Autodesk Inventor part; units mm, degrees
(part 2 of 2)
  spline S140 degree 2 poles (21.6159, 52.912) (21.6159, 52.7897) (21.701, 52.6195) (21.8632, 52.5397) (21.9616, 52.5397) knots 0 0 0 1 2 3 3 3
  spline S141 degree 2 poles (21.9616, 52.5397) (22.0308, 52.5397) (22.1611, 52.5849) (22.2675, 52.67) (22.3366, 52.7817) (22.3685, 52.8854) (22.3845, 52.9785) knots 0 0 0 1 2 3 4 5 5 5
  spline S142 degree 2 poles (52.1298, 59.6223) (52.0793, 59.0931) (52.0607, 58.7739) knots 0 0 0 1 1 1
  spline S143 degree 2 poles (52.0607, 58.7739) (52.0314, 58.3006) (52.0048, 57.548) knots 0 0 0 1 1 1
  spline S144 degree 2 poles (52.0048, 57.548) (51.9835, 56.9735) (51.9835, 56.7235) knots 0 0 0 1 1 1
  line L31 (51.9835, 56.7235) -> (51.9835, 56.4523)
  spline S145 degree 2 poles (51.9835, 56.4523) (51.7123, 56.4603) (51.5155, 56.4603) knots 0 0 0 1 1 1
  spline S146 degree 2 poles (51.5155, 56.4603) (51.324, 56.4603) (50.707, 56.439) (50.4358, 56.439) knots 0 0 0 1 2 2 2
  spline S147 degree 2 poles (50.4358, 56.439) (50.1246, 56.439) (49.6539, 56.5135) (49.247, 56.7448) (48.9731, 57.1198) (48.8295, 57.6251) (48.8295, 57.891) knots 0 0 0 1 2 3 4 5 5 5
  spline S148 degree 2 poles (48.8295, 57.891) (48.8295, 58.1543) (48.9412, 58.641) (49.1406, 59.0292) (49.4066, 59.3111) (49.5794, 59.4122) knots 0 0 0 1 2 3 4 4 4
  spline S149 degree 2 poles (49.5794, 59.4122) (49.7071, 59.484) (49.9677, 59.5691) (50.1938, 59.5957) knots 0 0 0 1 2 2 2
  spline S150 degree 2 poles (50.1938, 59.5957) (50.4438, 59.6223) (50.7629, 59.6223) knots 0 0 0 1 1 1
  line L32 (50.7629, 59.6223) -> (51.699, 59.6143)
  spline S151 degree 2 poles (51.699, 59.6143) (51.832, 59.6143) (52.1298, 59.6223) knots 0 0 0 1 1 1
  spline S152 degree 2 poles (51.1246, 58.9229) (50.9969, 58.9335) (50.8586, 58.9335) knots 0 0 0 1 1 1
  spline S153 degree 2 poles (50.8586, 58.9335) (50.6219, 58.9335) (50.2496, 58.8511) (49.9704, 58.5771) (49.8347, 58.1463) (49.8347, 57.9229) knots 0 0 0 1 2 3 4 4 4
  spline S154 degree 2 poles (49.8347, 57.9229) (49.8347, 57.6464) (50.0342, 57.2687) (50.3666, 57.1198) (50.6512, 57.1198) knots 0 0 0 1 2 3 3 3
  spline S155 degree 2 poles (50.6512, 57.1198) (50.8187, 57.1198) (51.0474, 57.1331) knots 0 0 0 1 1 1
  line L33 (51.0474, 57.1331) -> (51.1246, 58.9229)
  spline S156 degree 2 poles (46.1861, 58.9229) (46.2153, 59.0612) (46.3031, 59.5957) knots 0 0 0 1 1 1
  spline S157 degree 2 poles (46.3031, 59.5957) (46.5717, 59.6489) (46.9387, 59.6835) (47.1275, 59.6835) knots 0 0 0 1 2 2 2
  spline S158 degree 2 poles (47.1275, 59.6835) (47.4041, 59.6835) (47.8668, 59.6063) (48.2045, 59.4122) (48.4306, 59.1223) (48.5503, 58.7234) (48.5503, 58.5107) knots 0 0 0 1 2 3 4 5 5 5
  spline S159 degree 2 poles (48.5503, 58.5107) (48.5503, 58.2155) (48.3136, 57.6464) (47.9386, 57.3272) (47.4519, 57.1916) (47.1966, 57.1916) knots 0 0 0 1 2 3 4 4 4
  spline S160 degree 2 poles (47.1966, 57.1916) (46.9333, 57.1916) (46.452, 57.3139) (46.1169, 57.6198) (45.976, 58.0054) (45.976, 58.2288) knots 0 0 0 1 2 3 4 4 4
  spline S161 degree 2 poles (45.976, 58.2288) (45.976, 58.3617) (46.0052, 58.524) knots 0 0 0 1 1 1
  line L34 (46.0052, 58.524) -> (47.6328, 58.5266)
  spline S162 degree 2 poles (47.6328, 58.5266) (47.6354, 58.5639) (47.6354, 58.5931) knots 0 0 0 1 1 1
  spline S163 degree 2 poles (47.6354, 58.5931) (47.6354, 58.8431) (47.2764, 59.0798) (47.0211, 59.0798) knots 0 0 0 1 2 2 2
  spline S164 degree 2 poles (47.0211, 59.0798) (46.8669, 59.0798) (46.4733, 59.008) (46.1861, 58.9229) knots 0 0 0 1 2 2 2
  line L35 (47.6142, 58.1703) -> (46.8482, 58.1703)
  spline S165 degree 2 poles (46.8482, 58.1703) (46.8456, 58.1304) (46.8456, 58.1038) knots 0 0 0 1 1 1
  spline S166 degree 2 poles (46.8456, 58.1038) (46.8456, 57.9814) (46.9307, 57.8112) (47.0929, 57.7315) (47.1913, 57.7315) knots 0 0 0 1 2 3 3 3
  spline S167 degree 2 poles (47.1913, 57.7315) (47.2605, 57.7315) (47.3908, 57.7767) (47.4971, 57.8618) (47.5663, 57.9735) (47.5982, 58.0772) (47.6142, 58.1703) knots 0 0 0 1 2 3 4 5 5 5
  line L36 (45.0319, 59.6223) -> (45.2765, 58.8617)
  line L37 (45.2765, 58.8617) -> (45.8324, 57.2528)
  spline S168 degree 2 poles (45.8324, 57.2528) (45.5664, 57.2581) (45.3404, 57.2581) knots 0 0 0 1 1 1
  spline S169 degree 2 poles (45.3404, 57.2581) (45.1037, 57.2581) (44.8936, 57.2528) knots 0 0 0 1 1 1
  spline S170 degree 2 poles (44.8936, 57.2528) (44.8537, 57.4123) (44.6223, 58.2128) (44.4814, 58.766) knots 0 0 0 1 2 2 2
  line L38 (44.4814, 58.766) -> (44.4229, 58.5745)
  spline S171 degree 2 poles (44.4229, 58.5745) (44.4096, 58.5373) (44.3138, 58.2766) knots 0 0 0 1 1 1
  line L39 (44.3138, 58.2766) -> (43.9442, 57.2528)
  spline S172 degree 2 poles (43.9442, 57.2528) (43.6942, 57.2581) (43.4708, 57.2581) knots 0 0 0 1 1 1
  spline S173 degree 2 poles (43.4708, 57.2581) (43.2394, 57.2581) (42.9921, 57.2528) knots 0 0 0 1 1 1
  line L40 (42.9921, 57.2528) -> (43.3113, 57.9416)
  line L41 (43.3113, 57.9416) -> (43.9096, 59.3111)
  line L42 (43.9096, 59.3111) -> (44.0373, 59.6223)
  spline S174 degree 2 poles (44.0373, 59.6223) (44.3112, 59.617) (44.5213, 59.617) knots 0 0 0 1 1 1
  spline S175 degree 2 poles (44.5213, 59.617) (44.7473, 59.617) (45.0319, 59.6223) knots 0 0 0 1 1 1
  spline S176 degree 2 poles (40.5694, 58.9229) (40.5987, 59.0612) (40.6864, 59.5957) knots 0 0 0 1 1 1
  spline S177 degree 2 poles (40.6864, 59.5957) (40.955, 59.6489) (41.322, 59.6835) (41.5108, 59.6835) knots 0 0 0 1 2 2 2
  spline S178 degree 2 poles (41.5108, 59.6835) (41.7874, 59.6835) (42.2502, 59.6063) (42.5879, 59.4122) (42.8139, 59.1223) (42.9336, 58.7234) (42.9336, 58.5107) knots 0 0 0 1 2 3 4 5 5 5
  spline S179 degree 2 poles (42.9336, 58.5107) (42.9336, 58.2155) (42.6969, 57.6464) (42.322, 57.3272) (41.8353, 57.1916) (41.58, 57.1916) knots 0 0 0 1 2 3 4 4 4
  spline S180 degree 2 poles (41.58, 57.1916) (41.3167, 57.1916) (40.8354, 57.3139) (40.5003, 57.6198) (40.3593, 58.0054) (40.3593, 58.2288) knots 0 0 0 1 2 3 4 4 4
  spline S181 degree 2 poles (40.3593, 58.2288) (40.3593, 58.3617) (40.3886, 58.524) knots 0 0 0 1 1 1
  line L43 (40.3886, 58.524) -> (42.0161, 58.5266)
  spline S182 degree 2 poles (42.0161, 58.5266) (42.0188, 58.5639) (42.0188, 58.5931) knots 0 0 0 1 1 1
  spline S183 degree 2 poles (42.0188, 58.5931) (42.0188, 58.8431) (41.6598, 59.0798) (41.4045, 59.0798) knots 0 0 0 1 2 2 2
  spline S184 degree 2 poles (41.4045, 59.0798) (41.2502, 59.0798) (40.8566, 59.008) (40.5694, 58.9229) knots 0 0 0 1 2 2 2
  line L44 (41.9975, 58.1703) -> (41.2316, 58.1703)
  spline S185 degree 2 poles (41.2316, 58.1703) (41.2289, 58.1304) (41.2289, 58.1038) knots 0 0 0 1 1 1
  spline S186 degree 2 poles (41.2289, 58.1038) (41.2289, 57.9814) (41.314, 57.8112) (41.4763, 57.7315) (41.5747, 57.7315) knots 0 0 0 1 2 3 3 3
  spline S187 degree 2 poles (41.5747, 57.7315) (41.6438, 57.7315) (41.7741, 57.7767) (41.8805, 57.8618) (41.9496, 57.9735) (41.9816, 58.0772) (41.9975, 58.1703) knots 0 0 0 1 2 3 4 5 5 5
  line L45 (40.0588, 59.6223) -> (40.0163, 59.1223)
  line L46 (40.0163, 59.1223) -> (39.9285, 57.3857)
  line L47 (39.9285, 57.3857) -> (39.9019, 56.4523)
  spline S188 degree 2 poles (39.9019, 56.4523) (39.5801, 56.4576) (39.4179, 56.4576) knots 0 0 0 1 1 1
  spline S189 degree 2 poles (39.4179, 56.4576) (39.2051, 56.4576) (38.9498, 56.4523) knots 0 0 0 1 1 1
  line L48 (38.9498, 56.4523) -> (39.003, 57.165)
  line L49 (39.003, 57.165) -> (39.0881, 58.9202)
  line L50 (39.0881, 58.9202) -> (39.1067, 59.6223)
  spline S190 degree 2 poles (39.1067, 59.6223) (39.3541, 59.6196) (39.5535, 59.6196) knots 0 0 0 1 1 1
  line L51 (39.5535, 59.6196) -> (40.0588, 59.6223)
  spline S191 degree 2 poles (37.2, 57.1916) (36.9127, 57.1916) (36.3809, 57.3671) (36.0139, 57.6995) (35.8383, 58.1437) (35.8383, 58.399) knots 0 0 0 1 2 3 4 4 4
  spline S192 degree 2 poles (35.8383, 58.399) (35.8383, 58.649) (35.9953, 59.0957) (36.3649, 59.4893) (36.9393, 59.6835) (37.2611, 59.6835) knots 0 0 0 1 2 3 4 4 4
  spline S193 degree 2 poles (37.2611, 59.6835) (37.5537, 59.6835) (38.0988, 59.5106) (38.4632, 59.1808) (38.6467, 58.7208) (38.6467, 58.4681) knots 0 0 0 1 2 3 4 4 4
  spline S194 degree 2 poles (38.6467, 58.4681) (38.6467, 58.2155) (38.4685, 57.7554) (38.0802, 57.3884) (37.5084, 57.1916) (37.2, 57.1916) knots 0 0 0 1 2 3 4 4 4
  spline S195 degree 2 poles (37.2159, 57.8751) (37.3648, 57.8751) (37.5962, 58.0293) (37.7159, 58.3218) (37.7159, 58.4974) knots 0 0 0 1 2 3 3 3
  spline S196 degree 2 poles (37.7159, 58.4974) (37.7159, 58.7527) (37.4606, 59.0239) (37.2664, 59.0239) knots 0 0 0 1 2 2 2
  spline S197 degree 2 poles (37.2664, 59.0239) (37.1202, 59.0239) (36.8888, 58.8697) (36.7691, 58.5639) (36.7691, 58.391) knots 0 0 0 1 2 3 3 3
  spline S198 degree 2 poles (36.7691, 58.391) (36.7691, 58.2474) (36.8622, 58.0134) (37.075, 57.8751) (37.2159, 57.8751) knots 0 0 0 1 2 3 3 3
  spline S199 degree 2 poles (35.5644, 60.71) (35.5219, 60.234) (35.4926, 59.7606) knots 0 0 0 1 1 1
  spline S200 degree 2 poles (35.4926, 59.7606) (35.4394, 58.9495) (35.3995, 57.8511) (35.3995, 57.3113) knots 0 0 0 1 2 2 2
  spline S201 degree 2 poles (35.3995, 57.3113) (34.9288, 57.2395) (34.3943, 57.1916) (34.1284, 57.1916) knots 0 0 0 1 2 2 2
  spline S202 degree 2 poles (34.1284, 57.1916) (33.7933, 57.1916) (33.2295, 57.3299) (32.8891, 57.6836) (32.7162, 58.1729) (32.7162, 58.4389) knots 0 0 0 1 2 3 4 4 4
  spline S203 degree 2 poles (32.7162, 58.4389) (32.7162, 58.6835) (32.8545, 59.1409) (33.1444, 59.5079) (33.5167, 59.6835) (33.7454, 59.6835) knots 0 0 0 1 2 3 4 4 4
  spline S204 degree 2 poles (33.7454, 59.6835) (33.8598, 59.6835) (34.1044, 59.6382) (34.3225, 59.5558) (34.4688, 59.4707) (34.5778, 59.3883) knots 0 0 0 1 2 3 4 4 4
  line L52 (34.5778, 59.3883) -> (34.6017, 60.0372)
  spline S205 degree 2 poles (34.6017, 60.0372) (34.6203, 60.4813) (34.6203, 60.71) knots 0 0 0 1 1 1
  spline S206 degree 2 poles (34.6203, 60.71) (34.8889, 60.7047) (35.0804, 60.7047) knots 0 0 0 1 1 1
  spline S207 degree 2 poles (35.0804, 60.7047) (35.248, 60.7047) (35.5644, 60.71) knots 0 0 0 1 1 1
  spline S208 degree 2 poles (34.4954, 57.9043) (34.514, 58.008) (34.5273, 58.141) (34.5432, 58.3671) (34.5432, 58.4335) knots 0 0 0 1 2 3 3 3
  spline S209 degree 2 poles (34.5432, 58.4335) (34.5432, 58.625) (34.4235, 58.883) (34.2108, 59.0239) (34.0911, 59.0239) knots 0 0 0 1 2 3 3 3
  spline S210 degree 2 poles (34.0911, 59.0239) (33.9635, 59.0239) (33.7481, 58.8777) (33.6231, 58.5851) (33.6231, 58.4016) knots 0 0 0 1 2 3 3 3
  spline S211 degree 2 poles (33.6231, 58.4016) (33.6231, 58.1543) (33.8864, 57.8511) (34.1363, 57.8511) knots 0 0 0 1 2 2 2
  spline S212 degree 2 poles (34.1363, 57.8511) (34.2959, 57.8511) (34.4954, 57.9043) knots 0 0 0 1 1 1
  spline S213 degree 2 poles (30.0754, 58.9229) (30.1047, 59.0612) (30.1925, 59.5957) knots 0 0 0 1 1 1
  spline S214 degree 2 poles (30.1925, 59.5957) (30.461, 59.6489) (30.828, 59.6835) (31.0169, 59.6835) knots 0 0 0 1 2 2 2
  spline S215 degree 2 poles (31.0169, 59.6835) (31.2934, 59.6835) (31.7562, 59.6063) (32.0939, 59.4122) (32.32, 59.1223) (32.4396, 58.7234) (32.4396, 58.5107) knots 0 0 0 1 2 3 4 5 5 5
  spline S216 degree 2 poles (32.4396, 58.5107) (32.4396, 58.2155) (32.203, 57.6464) (31.828, 57.3272) (31.3413, 57.1916) (31.086, 57.1916) knots 0 0 0 1 2 3 4 4 4
  spline S217 degree 2 poles (31.086, 57.1916) (30.8227, 57.1916) (30.3414, 57.3139) (30.0063, 57.6198) (29.8653, 58.0054) (29.8653, 58.2288) knots 0 0 0 1 2 3 4 4 4
  spline S218 degree 2 poles (29.8653, 58.2288) (29.8653, 58.3617) (29.8946, 58.524) knots 0 0 0 1 1 1
  line L53 (29.8946, 58.524) -> (31.5221, 58.5266)
  spline S219 degree 2 poles (31.5221, 58.5266) (31.5248, 58.5639) (31.5248, 58.5931) knots 0 0 0 1 1 1
  spline S220 degree 2 poles (31.5248, 58.5931) (31.5248, 58.8431) (31.1658, 59.0798) (30.9105, 59.0798) knots 0 0 0 1 2 2 2
  spline S221 degree 2 poles (30.9105, 59.0798) (30.7562, 59.0798) (30.3627, 59.008) (30.0754, 58.9229) knots 0 0 0 1 2 2 2
  line L54 (31.5035, 58.1703) -> (30.7376, 58.1703)
  spline S222 degree 2 poles (30.7376, 58.1703) (30.735, 58.1304) (30.735, 58.1038) knots 0 0 0 1 1 1
  spline S223 degree 2 poles (30.735, 58.1038) (30.735, 57.9814) (30.8201, 57.8112) (30.9823, 57.7315) (31.0807, 57.7315) knots 0 0 0 1 2 3 3 3
  spline S224 degree 2 poles (31.0807, 57.7315) (31.1498, 57.7315) (31.2801, 57.7767) (31.3865, 57.8618) (31.4557, 57.9735) (31.4876, 58.0772) (31.5035, 58.1703) knots 0 0 0 1 2 3 4 5 5 5
  spline S225 degree 2 poles (26.9453, 59.6223) (27.1927, 59.617) (27.3575, 59.617) knots 0 0 0 1 1 1
  spline S226 degree 2 poles (27.3575, 59.617) (27.5437, 59.617) (27.8096, 59.6223) knots 0 0 0 1 1 1
  line L55 (27.8096, 59.6223) -> (27.7963, 59.3271)
  spline S227 degree 2 poles (27.7963, 59.3271) (27.8868, 59.4175) (28.0197, 59.5266) (28.2325, 59.6276) (28.4771, 59.6835) (28.6075, 59.6835) knots 0 0 0 1 2 3 4 4 4
  spline S228 degree 2 poles (28.6075, 59.6835) (28.8282, 59.6835) (29.2165, 59.5212) (29.4904, 59.2207) (29.626, 58.8112) (29.626, 58.5904) knots 0 0 0 1 2 3 4 4 4
  spline S229 degree 2 poles (29.626, 58.5904) (29.626, 58.2766) (29.3787, 57.6783) (28.9824, 57.3325) (28.4825, 57.1916) (28.1926, 57.1916) knots 0 0 0 1 2 3 4 4 4
  spline S230 degree 2 poles (28.1926, 57.1916) (27.9984, 57.1916) (27.7405, 57.2262) knots 0 0 0 1 1 1
  spline S231 degree 2 poles (27.7405, 57.2262) (27.7219, 56.9496) (27.7139, 56.4523) knots 0 0 0 1 1 1
  spline S232 degree 2 poles (27.7139, 56.4523) (27.4293, 56.4576) (27.2485, 56.4576) knots 0 0 0 1 1 1
  spline S233 degree 2 poles (27.2485, 56.4576) (27.0145, 56.4576) (26.7751, 56.4523) knots 0 0 0 1 1 1
  spline S234 degree 2 poles (26.7751, 56.4523) (26.8416, 57.1411) (26.9453, 59.1303) (26.9453, 59.6223) knots 0 0 0 1 2 2 2
  spline S235 degree 2 poles (27.7724, 57.8299) (27.8947, 57.8033) (28.0064, 57.8033) knots 0 0 0 1 1 1
  spline S236 degree 2 poles (28.0064, 57.8033) (28.2325, 57.8033) (28.5489, 57.9761) (28.7191, 58.3458) (28.7191, 58.524) knots 0 0 0 1 2 3 3 3
  spline S237 degree 2 poles (28.7191, 58.524) (28.7191, 58.6596) (28.6234, 58.875) (28.424, 59) (28.3043, 59) knots 0 0 0 1 2 3 3 3
  spline S238 degree 2 poles (28.3043, 59) (28.1766, 59) (27.9639, 58.8564) (27.8309, 58.5771) (27.7804, 58.1942) (27.7724, 57.8299) knots 0 0 0 1 2 3 4 4 4
  spline S239 degree 2 poles (25.246, 59.6223) (25.1821, 58.891) (25.0838, 56.9443) (25.0838, 56.4523) knots 0 0 0 1 2 2 2
  spline S240 degree 2 poles (25.0838, 56.4523) (24.8152, 56.4576) (24.5785, 56.4576) knots 0 0 0 1 1 1
  spline S241 degree 2 poles (24.5785, 56.4576) (24.3498, 56.4576) (24.129, 56.4523) knots 0 0 0 1 1 1
  spline S242 degree 2 poles (24.129, 56.4523) (24.1796, 56.814) (24.2035, 57.2501) knots 0 0 0 1 1 1
  spline S243 degree 2 poles (24.2035, 57.2501) (23.9907, 57.2155) (23.762, 57.1916) (23.653, 57.1916) knots 0 0 0 1 2 2 2
  spline S244 degree 2 poles (23.653, 57.1916) (23.294, 57.1916) (22.786, 57.4177) (22.4669, 57.9522) (22.4669, 58.3378) knots 0 0 0 1 2 3 3 3
  spline S245 degree 2 poles (22.4669, 58.3378) (22.4669, 58.7208) (22.7701, 59.3696) (23.2754, 59.6835) (23.6131, 59.6835) knots 0 0 0 1 2 3 3 3
  spline S246 degree 2 poles (23.6131, 59.6835) (23.7381, 59.6835) (23.9668, 59.6329) (24.1503, 59.5319) (24.278, 59.4202) (24.3577, 59.3271) knots 0 0 0 1 2 3 4 4 4
  line L56 (24.3577, 59.3271) -> (24.3684, 59.6223)
  spline S247 degree 2 poles (24.3684, 59.6223) (24.6157, 59.617) (24.7832, 59.617) knots 0 0 0 1 1 1
  spline S248 degree 2 poles (24.7832, 59.617) (24.9215, 59.617) (25.246, 59.6223) knots 0 0 0 1 1 1
  spline S249 degree 2 poles (24.2673, 57.9017) (24.2833, 58.2873) (24.2833, 58.3724) knots 0 0 0 1 1 1
  spline S250 degree 2 poles (24.2833, 58.3724) (24.2833, 58.5904) (24.2061, 58.8457) (23.9907, 59) (23.8551, 59) knots 0 0 0 1 2 3 3 3
  spline S251 degree 2 poles (23.8551, 59) (23.7168, 59) (23.5067, 58.8457) (23.3977, 58.5532) (23.3977, 58.3883) knots 0 0 0 1 2 3 3 3
  spline S252 degree 2 poles (23.3977, 58.3883) (23.3977, 58.1463) (23.661, 57.8511) (23.9083, 57.8511) knots 0 0 0 1 2 2 2
  spline S253 degree 2 poles (23.9083, 57.8511) (24.0625, 57.8511) (24.2673, 57.9017) knots 0 0 0 1 1 1
  spline S254 degree 2 poles (22.3153, 60.6834) (22.3871, 60.1302) (22.4137, 59.9946) knots 0 0 0 1 1 1
  spline S255 degree 2 poles (22.4137, 59.9946) (22.2675, 60.0637) (22.0414, 60.1143) (21.9616, 60.1143) knots 0 0 0 1 2 2 2
  spline S256 degree 2 poles (21.9616, 60.1143) (21.8739, 60.1143) (21.7249, 60.0691) (21.6345, 59.9999) (21.5308, 59.8616) (21.4803, 59.7606) (21.4537, 59.6675) knots 0 0 0 1 2 3 4 5 5 5
  line L57 (21.4537, 59.6675) -> (21.8898, 58.3484)
  line L58 (21.8898, 58.3484) -> (22.2648, 57.2528)
  spline S257 degree 2 poles (22.2648, 57.2528) (21.9191, 57.2581) (21.7808, 57.2581) knots 0 0 0 1 1 1
  spline S258 degree 2 poles (21.7808, 57.2581) (21.6159, 57.2581) (21.3367, 57.2528) knots 0 0 0 1 1 1
  spline S259 degree 2 poles (21.3367, 57.2528) (21.2915, 57.4309) (21.0521, 58.3085) (20.9989, 58.5559) knots 0 0 0 1 2 2 2
  spline S260 degree 2 poles (20.9989, 58.5559) (20.9697, 58.6942) (20.9404, 58.9043) knots 0 0 0 1 1 1
  line L59 (20.9404, 58.9043) -> (20.8925, 58.7208)
  spline S261 degree 2 poles (20.8925, 58.7208) (20.8686, 58.6463) (20.8101, 58.4548) (20.7622, 58.3218) knots 0 0 0 1 2 2 2
  line L60 (20.7622, 58.3218) -> (20.6106, 57.899)
  line L61 (20.6106, 57.899) -> (20.3607, 57.2528)
  spline S262 degree 2 poles (20.3607, 57.2528) (20.0708, 57.2581) (19.9219, 57.2581) knots 0 0 0 1 1 1
  spline S263 degree 2 poles (19.9219, 57.2581) (19.7916, 57.2581) (19.4565, 57.2528) knots 0 0 0 1 1 1
  line L62 (19.4565, 57.2528) -> (19.9059, 58.2633)
  line L63 (19.9059, 58.2633) -> (20.717, 60.1409)
  spline S264 degree 2 poles (20.717, 60.1409) (20.7941, 60.3004) (20.8659, 60.3935) knots 0 0 0 1 1 1
  spline S265 degree 2 poles (20.8659, 60.3935) (20.9351, 60.476) (21.0122, 60.5398) knots 0 0 0 1 1 1
  spline S266 degree 2 poles (21.0122, 60.5398) (21.0867, 60.5983) (21.1744, 60.6355) knots 0 0 0 1 1 1
  spline S267 degree 2 poles (21.1744, 60.6355) (21.2888, 60.6887) (21.4297, 60.7206) knots 0 0 0 1 1 1
  spline S268 degree 2 poles (21.4297, 60.7206) (21.5813, 60.7525) (21.7409, 60.7525) knots 0 0 0 1 1 1
  spline S269 degree 2 poles (21.7409, 60.7525) (21.8127, 60.7525) (22.0494, 60.7313) (22.1956, 60.71) (22.3153, 60.6834) knots 0 0 0 1 2 3 3 3
  spline S270 degree 2 poles (19.2889, 59.6223) (19.2703, 59.3111) (19.257, 58.7819) knots 0 0 0 1 1 1
  line L64 (19.257, 58.7819) -> (18.7783, 58.7899)
  spline S271 degree 2 poles (18.7783, 58.7899) (18.7012, 58.7899) (18.3741, 58.7819) knots 0 0 0 1 1 1
  spline S272 degree 2 poles (18.3741, 58.7819) (18.3927, 59.0346) (18.4166, 59.6223) knots 0 0 0 1 1 1
  line L65 (18.4166, 59.6223) -> (18.8209, 59.617)
  spline S273 degree 2 poles (18.8209, 59.617) (18.8634, 59.617) (19.2889, 59.6223) knots 0 0 0 1 1 1
  spline S274 degree 2 poles (19.2331, 58.0931) (19.2118, 57.7208) (19.1985, 57.2528) knots 0 0 0 1 1 1
  line L66 (19.1985, 57.2528) -> (18.7225, 57.2581)
  spline S275 degree 2 poles (18.7225, 57.2581) (18.6454, 57.2581) (18.3182, 57.2528) knots 0 0 0 1 1 1
  spline S276 degree 2 poles (18.3182, 57.2528) (18.3342, 57.4788) (18.3608, 58.0931) knots 0 0 0 1 1 1
  line L67 (18.3608, 58.0931) -> (18.765, 58.0852)
  spline S277 degree 2 poles (18.765, 58.0852) (18.8076, 58.0852) (19.2331, 58.0931) knots 0 0 0 1 1 1
  spline S278 degree 2 poles (50.1326, 63.1972) (50.1326, 63.3753) (50.3081, 63.6865) (50.614, 63.862) (50.7868, 63.862) knots 0 0 0 1 2 3 3 3
  spline S279 degree 2 poles (50.7868, 63.862) (50.9597, 63.862) (51.2655, 63.6838) (51.441, 63.3727) (51.441, 63.1972) knots 0 0 0 1 2 3 3 3
  spline S280 degree 2 poles (51.441, 63.1972) (51.441, 63.0216) (51.2655, 62.7131) (50.9597, 62.535) (50.7815, 62.535) knots 0 0 0 1 2 3 3 3
  spline S281 degree 2 poles (50.7815, 62.535) (50.6113, 62.535) (50.3081, 62.7105) (50.1326, 63.019) (50.1326, 63.1972) knots 0 0 0 1 2 3 3 3
  line L68 (43.04, 64.8141) -> (42.8485, 64.479)
  line L69 (42.8485, 64.479) -> (41.6465, 62.2185)
  line L70 (41.6465, 62.2185) -> (41.5188, 61.9659)
  spline S282 degree 2 poles (41.5188, 61.9659) (41.463, 61.8542) (41.3646, 61.6441) knots 0 0 0 1 1 1
  spline S283 degree 2 poles (41.3646, 61.6441) (40.955, 61.6494) (40.7662, 61.6494) knots 0 0 0 1 1 1
  spline S284 degree 2 poles (40.7662, 61.6494) (40.4391, 61.6494) (40.1599, 61.6441) knots 0 0 0 1 1 1
  line L71 (40.1599, 61.6441) -> (39.8221, 62.6121)
  line L72 (39.8221, 62.6121) -> (39.1333, 64.4737)
  line L73 (39.1333, 64.4737) -> (38.9977, 64.8141)
  spline S285 degree 2 poles (38.9977, 64.8141) (39.3993, 64.8087) (39.4844, 64.8087) knots 0 0 0 1 1 1
  spline S286 degree 2 poles (39.4844, 64.8087) (39.6812, 64.8087) (40.0588, 64.8141) knots 0 0 0 1 1 1
  spline S287 degree 2 poles (40.0588, 64.8141) (40.1599, 64.4311) (40.354, 63.9125) knots 0 0 0 1 1 1
  line L74 (40.354, 63.9125) -> (41.5241, 63.9125)
  spline S288 degree 2 poles (41.5241, 63.9125) (41.7236, 64.3221) (41.9417, 64.8141) knots 0 0 0 1 1 1
  spline S289 degree 2 poles (41.9417, 64.8141) (42.3725, 64.8087) (42.4709, 64.8087) knots 0 0 0 1 1 1
  spline S290 degree 2 poles (42.4709, 64.8087) (42.6464, 64.8087) (43.04, 64.8141) knots 0 0 0 1 1 1
  line L75 (41.2422, 63.237) -> (40.5215, 63.237)
  spline S291 degree 2 poles (40.5215, 63.237) (40.7901, 62.418) (40.8141, 62.3355) knots 0 0 0 1 1 1
  spline S292 degree 2 poles (40.8141, 62.3355) (40.9683, 62.6759) (41.0747, 62.894) knots 0 0 0 1 1 1
  line L76 (41.0747, 62.894) -> (41.2422, 63.237)
  line L77 (38.7876, 64.8141) -> (38.7451, 64.3141)
  line L78 (38.7451, 64.3141) -> (38.6573, 62.5775)
  line L79 (38.6573, 62.5775) -> (38.6307, 61.6441)
  spline S293 degree 2 poles (38.6307, 61.6441) (38.3089, 61.6494) (38.1467, 61.6494) knots 0 0 0 1 1 1
  spline S294 degree 2 poles (38.1467, 61.6494) (37.934, 61.6494) (37.6786, 61.6441) knots 0 0 0 1 1 1
  line L80 (37.6786, 61.6441) -> (37.7318, 62.3568)
  line L81 (37.7318, 62.3568) -> (37.8169, 64.112)
  line L82 (37.8169, 64.112) -> (37.8356, 64.8141)
  spline S295 degree 2 poles (37.8356, 64.8141) (38.0829, 64.8114) (38.2823, 64.8114) knots 0 0 0 1 1 1
  line L83 (38.2823, 64.8114) -> (38.7876, 64.8141)
  spline S296 degree 2 poles (37.2053, 64.8141) (37.1601, 64.3673) (37.0989, 63.1094) knots 0 0 0 1 1 1
  line L84 (37.0989, 63.1094) -> (37.3808, 63.1094)
  spline S297 degree 2 poles (37.3808, 63.1094) (37.3728, 63.0376) (37.3489, 62.5669) (37.3462, 62.4632) knots 0 0 0 1 2 2 2
  line L85 (37.3462, 62.4632) -> (37.0191, 62.4632)
  spline S298 degree 2 poles (37.0191, 62.4632) (37.0218, 62.3701) (37.0218, 62.3036) knots 0 0 0 1 1 1
  spline S299 degree 2 poles (37.0218, 62.3036) (37.0218, 62.0908) (36.9766, 61.8488) (36.8596, 61.6786) (36.6441, 61.5457) (36.3702, 61.5005) (36.224, 61.5005) knots 0 0 0 1 2 3 4 5 5 5
  spline S300 degree 2 poles (36.224, 61.5005) (36.091, 61.5005) (35.7772, 61.535) (35.5565, 61.5935) knots 0 0 0 1 2 2 2
  spline S301 degree 2 poles (35.5565, 61.5935) (35.5511, 61.9632) (35.5272, 62.2052) knots 0 0 0 1 1 1
  spline S302 degree 2 poles (35.5272, 62.2052) (35.7586, 62.1228) (35.9421, 62.1228) knots 0 0 0 1 1 1
  spline S303 degree 2 poles (35.9421, 62.1228) (36.0671, 62.1228) (36.2107, 62.2398) (36.2107, 62.394) knots 0 0 0 1 2 2 2
  line L86 (36.2107, 62.394) -> (36.208, 62.4632)
  line L87 (36.208, 62.4632) -> (35.6708, 62.4632)
  spline S304 degree 2 poles (35.6708, 62.4632) (35.6894, 62.7318) (35.708, 63.1094) knots 0 0 0 1 1 1
  line L88 (35.708, 63.1094) -> (36.1894, 63.1094)
  line L89 (36.1894, 63.1094) -> (36.2665, 64.8141)
  spline S305 degree 2 poles (36.2665, 64.8141) (36.5431, 64.8087) (36.7399, 64.8087) knots 0 0 0 1 1 1
  spline S306 degree 2 poles (36.7399, 64.8087) (36.9393, 64.8087) (37.2053, 64.8141) knots 0 0 0 1 1 1
  spline S307 degree 2 poles (35.2081, 63.12) (35.1629, 62.8887) (35.1416, 62.7158) (35.115, 62.5296) knots 0 0 0 1 2 2 2
  spline S308 degree 2 poles (35.115, 62.5296) (34.4475, 62.3834) (33.9661, 62.3834) knots 0 0 0 1 1 1
  spline S309 degree 2 poles (33.9661, 62.3834) (33.6922, 62.3834) (33.2375, 62.5057) (32.9822, 62.7796) (32.9822, 63.0349) knots 0 0 0 1 2 3 3 3
  spline S310 degree 2 poles (32.9822, 63.0349) (32.9822, 63.1652) (33.0513, 64.0748) (33.0699, 64.8141) knots 0 0 0 1 2 2 2
  spline S311 degree 2 poles (33.0699, 64.8141) (33.296, 64.8087) (33.522, 64.8087) knots 0 0 0 1 1 1
  spline S312 degree 2 poles (33.522, 64.8087) (33.7401, 64.8087) (33.9874, 64.8141) knots 0 0 0 1 1 1
  spline S313 degree 2 poles (33.9874, 64.8141) (33.9555, 64.5588) (33.9156, 63.7609) knots 0 0 0 1 1 1
  spline S314 degree 2 poles (33.9156, 63.7609) (34.0034, 63.8035) (34.1044, 63.8407) (34.3544, 63.9152) (34.4954, 63.9657) (34.5991, 64.0455) (34.6443, 64.1279) (34.6443, 64.1785) knots 0 0 0 1 2 3 4 5 6 6 6
  spline S315 degree 2 poles (34.6443, 64.1785) (34.6443, 64.2583) (34.5193, 64.3699) (34.3837, 64.3699) knots 0 0 0 1 2 2 2
  spline S316 degree 2 poles (34.3837, 64.3699) (34.3331, 64.3699) (34.2241, 64.354) (34.1257, 64.3221) knots 0 0 0 1 2 2 2
  spline S317 degree 2 poles (34.1257, 64.3221) (34.1922, 64.5003) (34.2853, 64.8433) knots 0 0 0 1 1 1
  spline S318 degree 2 poles (34.2853, 64.8433) (34.4847, 64.8752) (34.6629, 64.8752) knots 0 0 0 1 1 1
  spline S319 degree 2 poles (34.6629, 64.8752) (34.9501, 64.8752) (35.3331, 64.7157) (35.5405, 64.3566) (35.5405, 64.1785) knots 0 0 0 1 2 3 3 3
  spline S320 degree 2 poles (35.5405, 64.1785) (35.5405, 64.0694) (35.4634, 63.8593) (35.3011, 63.6599) (35.0831, 63.5189) (34.7054, 63.3939) (34.4156, 63.3381) knots 0 0 0 1 2 3 4 5 5 5
  spline S321 degree 2 poles (34.4156, 63.3381) (34.2932, 63.3142) (34.0911, 63.261) (34.006, 63.2211) (33.9528, 63.1679) (33.9289, 63.1094) (33.9289, 63.0775) knots 0 0 0 1 2 3 4 5 5 5
  spline S322 degree 2 poles (33.9289, 63.0775) (33.9289, 62.9897) (34.0778, 62.894) (34.2214, 62.894) knots 0 0 0 1 2 2 2
  spline S323 degree 2 poles (34.2214, 62.894) (34.6203, 62.894) (35.2081, 63.12) knots 0 0 0 1 1 1
  spline S324 degree 2 poles (32.57, 64.8141) (32.5035, 64.2875) (32.4317, 63.0137) (32.4237, 62.4445) knots 0 0 0 1 2 2 2
  spline S325 degree 2 poles (32.4237, 62.4445) (32.1471, 62.4499) (31.945, 62.4499) knots 0 0 0 1 1 1
  spline S326 degree 2 poles (31.945, 62.4499) (31.7083, 62.4499) (31.4929, 62.4445) knots 0 0 0 1 1 1
  line L90 (31.4929, 62.4445) -> (31.5168, 62.761)
  spline S327 degree 2 poles (31.5168, 62.761) (31.4397, 62.6733) (31.328, 62.5749) (31.1631, 62.4791) (30.977, 62.418) (30.7562, 62.3834) (30.6366, 62.3834) knots 0 0 0 1 2 3 4 5 5 5
  spline S328 degree 2 poles (30.6366, 62.3834) (30.469, 62.3834) (30.1499, 62.4552) (29.9371, 62.5882) (29.7909, 62.7849) (29.7457, 63.0137) (29.7457, 63.1333) knots 0 0 0 1 2 3 4 5 5 5
  spline S329 degree 2 poles (29.7457, 63.1333) (29.7457, 63.2211) (29.7643, 63.5136) knots 0 0 0 1 1 1
  line L91 (29.7643, 63.5136) -> (29.8042, 64.354)
  spline S330 degree 2 poles (29.8042, 64.354) (29.8148, 64.604) (29.8148, 64.8141) knots 0 0 0 1 1 1
  spline S331 degree 2 poles (29.8148, 64.8141) (30.0515, 64.8087) (30.2536, 64.8087) knots 0 0 0 1 1 1
  spline S332 degree 2 poles (30.2536, 64.8087) (30.5302, 64.8087) (30.7589, 64.8141) knots 0 0 0 1 1 1
  spline S333 degree 2 poles (30.7589, 64.8141) (30.7376, 64.604) (30.6924, 63.7689) (30.6924, 63.6014) knots 0 0 0 1 2 2 2
  spline S334 degree 2 poles (30.6924, 63.6014) (30.6924, 63.3381) (30.8945, 63.1307) (31.0461, 63.1307) knots 0 0 0 1 2 2 2
  spline S335 degree 2 poles (31.0461, 63.1307) (31.1817, 63.1307) (31.4211, 63.3062) (31.5514, 63.6439) (31.6046, 64.4152) (31.6126, 64.8141) knots 0 0 0 1 2 3 4 4 4
  spline S336 degree 2 poles (31.6126, 64.8141) (31.8466, 64.8087) (32.0673, 64.8087) knots 0 0 0 1 1 1
  spline S337 degree 2 poles (32.0673, 64.8087) (32.2987, 64.8087) (32.57, 64.8141) knots 0 0 0 1 1 1
  spline S338 degree 2 poles (27.9346, 62.3834) (27.6474, 62.3834) (27.1155, 62.5589) (26.7485, 62.8913) (26.573, 63.3354) (26.573, 63.5907) knots 0 0 0 1 2 3 4 4 4
  spline S339 degree 2 poles (26.573, 63.5907) (26.573, 63.8407) (26.7299, 64.2875) (27.0996, 64.6811) (27.674, 64.8752) (27.9958, 64.8752) knots 0 0 0 1 2 3 4 4 4
  spline S340 degree 2 poles (27.9958, 64.8752) (28.2883, 64.8752) (28.8335, 64.7024) (29.1978, 64.3726) (29.3813, 63.9125) (29.3813, 63.6599) knots 0 0 0 1 2 3 4 4 4
  spline S341 degree 2 poles (29.3813, 63.6599) (29.3813, 63.4072) (29.2032, 62.9472) (28.8149, 62.5802) (28.2431, 62.3834) (27.9346, 62.3834) knots 0 0 0 1 2 3 4 4 4
  spline S342 degree 2 poles (27.9506, 63.0668) (28.0995, 63.0668) (28.3309, 63.2211) (28.4505, 63.5136) (28.4505, 63.6891) knots 0 0 0 1 2 3 3 3
  spline S343 degree 2 poles (28.4505, 63.6891) (28.4505, 63.9444) (28.1952, 64.2157) (28.0011, 64.2157) knots 0 0 0 1 2 2 2
  spline S344 degree 2 poles (28.0011, 64.2157) (27.8548, 64.2157) (27.6235, 64.0615) (27.5038, 63.7556) (27.5038, 63.5828) knots 0 0 0 1 2 3 3 3
  spline S345 degree 2 poles (27.5038, 63.5828) (27.5038, 63.4392) (27.5969, 63.2051) (27.8096, 63.0668) (27.9506, 63.0668) knots 0 0 0 1 2 3 3 3
  spline S346 degree 2 poles (25.0173, 64.8141) (24.9588, 64.2157) (24.9056, 63.4072) (24.8524, 62.0669) (24.8524, 61.8488) knots 0 0 0 1 2 3 3 3
  line L92 (24.8524, 61.8488) -> (24.855, 61.6441)
  spline S347 degree 2 poles (24.855, 61.6441) (24.3072, 61.6494) (23.528, 61.6494) knots 0 0 0 1 1 1
  spline S348 degree 2 poles (23.528, 61.6494) (22.81, 61.6494) (22.2621, 61.6441) knots 0 0 0 1 1 1
  line L93 (22.2621, 61.6441) -> (22.2675, 61.7212)
  spline S349 degree 2 poles (22.2675, 61.7212) (22.2701, 61.7478) (22.2781, 61.9206) knots 0 0 0 1 1 1
  line L94 (22.2781, 61.9206) -> (22.2914, 62.1733)
  spline S350 degree 2 poles (22.2914, 62.1733) (22.2967, 62.2531) (22.2967, 62.3382) knots 0 0 0 1 1 1
  spline S351 degree 2 poles (22.2967, 62.3382) (22.7461, 62.3196) (23.0493, 62.3196) knots 0 0 0 1 1 1
  spline S352 degree 2 poles (23.0493, 62.3196) (23.3844, 62.3196) (23.6184, 62.3222) (23.8684, 62.3302) knots 0 0 0 1 2 2 2
  line L95 (23.8684, 62.3302) -> (23.8977, 62.8647)
  spline S353 degree 2 poles (23.8977, 62.8647) (23.6237, 62.8727) (23.2567, 62.8727) knots 0 0 0 1 1 1
  spline S354 degree 2 poles (23.2567, 62.8727) (23.1264, 62.8727) (22.5653, 62.8541) knots 0 0 0 1 1 1
  spline S355 degree 2 poles (22.5653, 62.8541) (22.5892, 63.1519) (22.6105, 63.5641) knots 0 0 0 1 1 1
  spline S356 degree 2 poles (22.6105, 63.5641) (23.0121, 63.5588) (23.2275, 63.5588) knots 0 0 0 1 1 1
  spline S357 degree 2 poles (23.2275, 63.5588) (23.5493, 63.5588) (23.9455, 63.5748) knots 0 0 0 1 1 1
  line L96 (23.9455, 63.5748) -> (23.9748, 64.1412)
  line L97 (23.9748, 64.1412) -> (23.7062, 64.1412)
  spline S358 degree 2 poles (23.7062, 64.1412) (23.5865, 64.1412) (23.2169, 64.1333) knots 0 0 0 1 1 1
  line L98 (23.2169, 64.1333) -> (22.7355, 64.1226)
  spline S359 degree 2 poles (22.7355, 64.1226) (22.6265, 64.12) (22.3765, 64.104) knots 0 0 0 1 1 1
  spline S360 degree 2 poles (22.3765, 64.104) (22.4031, 64.4471) (22.4217, 64.8141) knots 0 0 0 1 1 1
  spline S361 degree 2 poles (22.4217, 64.8141) (22.9908, 64.8087) (23.6663, 64.8087) knots 0 0 0 1 1 1
  line L99 (23.6663, 64.8087) -> (24.6875, 64.8114)
  line L100 (24.6875, 64.8114) -> (25.0173, 64.8141)
  line L101 (21.9005, 64.8141) -> (21.8366, 63.6945)
  line L102 (21.8366, 63.6945) -> (21.7994, 62.8195)
  line L103 (21.7994, 62.8195) -> (21.7941, 62.4445)
  spline S362 degree 2 poles (21.7941, 62.4445) (21.5388, 62.4499) (21.3446, 62.4499) knots 0 0 0 1 1 1
  spline S363 degree 2 poles (21.3446, 62.4499) (21.1239, 62.4499) (20.9138, 62.4445) knots 0 0 0 1 1 1
  line L104 (20.9138, 62.4445) -> (20.9324, 62.753)
  spline S364 degree 2 poles (20.9324, 62.753) (20.858, 62.66) (20.7596, 62.5589) (20.616, 62.4685) (20.4617, 62.4153) (20.2702, 62.3834) (20.1665, 62.3834) knots 0 0 0 1 2 3 4 5 5 5
  spline S365 degree 2 poles (20.1665, 62.3834) (20.0469, 62.3834) (19.8474, 62.4233) (19.7038, 62.4844) (19.5974, 62.5616) (19.515, 62.6626) (19.4618, 62.7584) knots 0 0 0 1 2 3 4 5 5 5
  spline S366 degree 2 poles (19.4618, 62.7584) (19.3607, 62.6094) (19.132, 62.4552) (18.8421, 62.3834) (18.6879, 62.3834) knots 0 0 0 1 2 3 3 3
  spline S367 degree 2 poles (18.6879, 62.3834) (18.4858, 62.3834) (18.1268, 62.5004) (17.8981, 62.7849) (17.8981, 63.0137) knots 0 0 0 1 2 3 3 3
  spline S368 degree 2 poles (17.8981, 63.0137) (17.8981, 63.12) (17.9273, 63.5509) (17.9832, 64.604) (17.9858, 64.8141) knots 0 0 0 1 2 3 3 3
  spline S369 degree 2 poles (17.9858, 64.8141) (18.1986, 64.8087) (18.398, 64.8087) knots 0 0 0 1 1 1
  spline S370 degree 2 poles (18.398, 64.8087) (18.6427, 64.8087) (18.9086, 64.8141) knots 0 0 0 1 1 1
  spline S371 degree 2 poles (18.9086, 64.8141) (18.8847, 64.5189) (18.8342, 63.6306) (18.8342, 63.4578) knots 0 0 0 1 2 2 2
  spline S372 degree 2 poles (18.8342, 63.4578) (18.8342, 63.3088) (18.906, 63.1599) (19.015, 63.1067) (19.0788, 63.1067) knots 0 0 0 1 2 3 3 3
  spline S373 degree 2 poles (19.0788, 63.1067) (19.148, 63.1067) (19.1985, 63.1333) knots 0 0 0 1 1 1
  spline S374 degree 2 poles (19.1985, 63.1333) (19.2544, 63.1599) (19.2969, 63.2184) knots 0 0 0 1 1 1
  spline S375 degree 2 poles (19.2969, 63.2184) (19.3528, 63.2956) (19.3873, 63.4126) knots 0 0 0 1 1 1
  spline S376 degree 2 poles (19.3873, 63.4126) (19.4139, 63.503) (19.4299, 63.6891) knots 0 0 0 1 1 1
  spline S377 degree 2 poles (19.4299, 63.6891) (19.4485, 63.8806) (19.4565, 64.1918) knots 0 0 0 1 1 1
  line L105 (19.4565, 64.1918) -> (19.4751, 64.8141)
  spline S378 degree 2 poles (19.4751, 64.8141) (19.7251, 64.8087) (19.9245, 64.8087) knots 0 0 0 1 1 1
  spline S379 degree 2 poles (19.9245, 64.8087) (20.1293, 64.8087) (20.4059, 64.8141) knots 0 0 0 1 1 1
  spline S380 degree 2 poles (20.4059, 64.8141) (20.3846, 64.6066) (20.3314, 63.6333) (20.3314, 63.4684) knots 0 0 0 1 2 2 2
  spline S381 degree 2 poles (20.3314, 63.4684) (20.3314, 63.3275) (20.3873, 63.1892) (20.4857, 63.1067) (20.5708, 63.1067) knots 0 0 0 1 2 3 3 3
  spline S382 degree 2 poles (20.5708, 63.1067) (20.6612, 63.1067) (20.7941, 63.2131) (20.8899, 63.4126) (20.9298, 63.7636) (20.9617, 64.4816) (20.967, 64.8141) knots 0 0 0 1 2 3 4 5 5 5
  spline S383 degree 2 poles (20.967, 64.8141) (21.2462, 64.8087) (21.4218, 64.8087) knots 0 0 0 1 1 1
  spline S384 degree 2 poles (21.4218, 64.8087) (21.6132, 64.8087) (21.9005, 64.8141) knots 0 0 0 1 1 1
  spline S385 degree 2 poles (17.2545, 63.12) (17.2093, 62.8887) (17.188, 62.7158) (17.1614, 62.5296) knots 0 0 0 1 2 2 2
  spline S386 degree 2 poles (17.1614, 62.5296) (16.4939, 62.3834) (16.0126, 62.3834) knots 0 0 0 1 1 1
  spline S387 degree 2 poles (16.0126, 62.3834) (15.7386, 62.3834) (15.2839, 62.5057) (15.0286, 62.7796) (15.0286, 63.0349) knots 0 0 0 1 2 3 3 3
  spline S388 degree 2 poles (15.0286, 63.0349) (15.0286, 63.1652) (15.0977, 64.0748) (15.1163, 64.8141) knots 0 0 0 1 2 2 2
  spline S389 degree 2 poles (15.1163, 64.8141) (15.3424, 64.8087) (15.5684, 64.8087) knots 0 0 0 1 1 1
  spline S390 degree 2 poles (15.5684, 64.8087) (15.7865, 64.8087) (16.0338, 64.8141) knots 0 0 0 1 1 1
  spline S391 degree 2 poles (16.0338, 64.8141) (16.0019, 64.5588) (15.962, 63.7609) knots 0 0 0 1 1 1
  spline S392 degree 2 poles (15.962, 63.7609) (16.0498, 63.8035) (16.1508, 63.8407) (16.4008, 63.9152) (16.5418, 63.9657) (16.6455, 64.0455) (16.6907, 64.1279) (16.6907, 64.1785) knots 0 0 0 1 2 3 4 5 6 6 6
  spline S393 degree 2 poles (16.6907, 64.1785) (16.6907, 64.2583) (16.5657, 64.3699) (16.4301, 64.3699) knots 0 0 0 1 2 2 2
  spline S394 degree 2 poles (16.4301, 64.3699) (16.3795, 64.3699) (16.2705, 64.354) (16.1721, 64.3221) knots 0 0 0 1 2 2 2
  spline S395 degree 2 poles (16.1721, 64.3221) (16.2386, 64.5003) (16.3317, 64.8433) knots 0 0 0 1 1 1
  spline S396 degree 2 poles (16.3317, 64.8433) (16.5311, 64.8752) (16.7093, 64.8752) knots 0 0 0 1 1 1
  spline S397 degree 2 poles (16.7093, 64.8752) (16.9965, 64.8752) (17.3795, 64.7157) (17.5869, 64.3566) (17.5869, 64.1785) knots 0 0 0 1 2 3 3 3
  spline S398 degree 2 poles (17.5869, 64.1785) (17.5869, 64.0694) (17.5098, 63.8593) (17.3476, 63.6599) (17.1295, 63.5189) (16.7519, 63.3939) (16.462, 63.3381) knots 0 0 0 1 2 3 4 5 5 5
  spline S399 degree 2 poles (16.462, 63.3381) (16.3397, 63.3142) (16.1375, 63.261) (16.0524, 63.2211) (15.9993, 63.1679) (15.9753, 63.1094) (15.9753, 63.0775) knots 0 0 0 1 2 3 4 5 5 5
  spline S400 degree 2 poles (15.9753, 63.0775) (15.9753, 62.9897) (16.1242, 62.894) (16.2679, 62.894) knots 0 0 0 1 2 2 2
  spline S401 degree 2 poles (16.2679, 62.894) (16.6668, 62.894) (17.2545, 63.12) knots 0 0 0 1 1 1
  spline S402 degree 2 poles (14.6164, 64.8141) (14.5499, 64.2875) (14.4781, 63.0137) (14.4701, 62.4445) knots 0 0 0 1 2 2 2
  spline S403 degree 2 poles (14.4701, 62.4445) (14.1935, 62.4499) (13.9914, 62.4499) knots 0 0 0 1 1 1
  spline S404 degree 2 poles (13.9914, 62.4499) (13.7547, 62.4499) (13.5393, 62.4445) knots 0 0 0 1 1 1
  line L106 (13.5393, 62.4445) -> (13.5632, 62.761)
  spline S405 degree 2 poles (13.5632, 62.761) (13.4861, 62.6733) (13.3744, 62.5749) (13.2095, 62.4791) (13.0234, 62.418) (12.8027, 62.3834) (12.683, 62.3834) knots 0 0 0 1 2 3 4 5 5 5
  spline S406 degree 2 poles (12.683, 62.3834) (12.5154, 62.3834) (12.1963, 62.4552) (11.9836, 62.5882) (11.8373, 62.7849) (11.7921, 63.0137) (11.7921, 63.1333) knots 0 0 0 1 2 3 4 5 5 5
  spline S407 degree 2 poles (11.7921, 63.1333) (11.7921, 63.2211) (11.8107, 63.5136) knots 0 0 0 1 1 1
  line L107 (11.8107, 63.5136) -> (11.8506, 64.354)
  spline S408 degree 2 poles (11.8506, 64.354) (11.8612, 64.604) (11.8612, 64.8141) knots 0 0 0 1 1 1
  spline S409 degree 2 poles (11.8612, 64.8141) (12.0979, 64.8087) (12.3, 64.8087) knots 0 0 0 1 1 1
  spline S410 degree 2 poles (12.3, 64.8087) (12.5766, 64.8087) (12.8053, 64.8141) knots 0 0 0 1 1 1
  spline S411 degree 2 poles (12.8053, 64.8141) (12.784, 64.604) (12.7388, 63.7689) (12.7388, 63.6014) knots 0 0 0 1 2 2 2
  spline S412 degree 2 poles (12.7388, 63.6014) (12.7388, 63.3381) (12.9409, 63.1307) (13.0925, 63.1307) knots 0 0 0 1 2 2 2
  spline S413 degree 2 poles (13.0925, 63.1307) (13.2282, 63.1307) (13.4675, 63.3062) (13.5978, 63.6439) (13.651, 64.4152) (13.659, 64.8141) knots 0 0 0 1 2 3 4 4 4
  spline S414 degree 2 poles (13.659, 64.8141) (13.893, 64.8087) (14.1137, 64.8087) knots 0 0 0 1 1 1
  spline S415 degree 2 poles (14.1137, 64.8087) (14.3451, 64.8087) (14.6164, 64.8141) knots 0 0 0 1 1 1
  spline S416 degree 2 poles (8.763, 64.8141) (9.0263, 64.8087) (9.2045, 64.8087) knots 0 0 0 1 1 1
  spline S417 degree 2 poles (9.2045, 64.8087) (9.4226, 64.8087) (9.6433, 64.8141) knots 0 0 0 1 1 1
  line L108 (9.6433, 64.8141) -> (9.646, 64.4949)
  spline S418 degree 2 poles (9.646, 64.4949) (9.7284, 64.6013) (9.8454, 64.705) (9.981, 64.7848) (10.1512, 64.8433) (10.372, 64.8752) (10.4863, 64.8752) knots 0 0 0 1 2 3 4 5 5 5
  spline S419 degree 2 poles (10.4863, 64.8752) (10.6698, 64.8752) (10.9969, 64.7901) (11.2469, 64.5854) (11.3373, 64.3247) (11.3373, 64.1519) knots 0 0 0 1 2 3 4 4 4
  spline S420 degree 2 poles (11.3373, 64.1519) (11.3373, 64.112) (11.3294, 64.0216) knots 0 0 0 1 1 1
  line L109 (11.3294, 64.0216) -> (11.2948, 63.495)
  spline S421 degree 2 poles (11.2948, 63.495) (11.2788, 63.2051) (11.2629, 62.8541) knots 0 0 0 1 1 1
  spline S422 degree 2 poles (11.2629, 62.8541) (11.2549, 62.636) (11.2549, 62.4445) knots 0 0 0 1 1 1
  spline S423 degree 2 poles (11.2549, 62.4445) (10.9677, 62.4499) (10.7656, 62.4499) knots 0 0 0 1 1 1
  spline S424 degree 2 poles (10.7656, 62.4499) (10.5608, 62.4499) (10.3135, 62.4445) knots 0 0 0 1 1 1
  line L110 (10.3135, 62.4445) -> (10.3853, 63.3275)
  spline S425 degree 2 poles (10.3853, 63.3275) (10.4012, 63.5296) (10.4039, 63.6758) (10.4039, 63.7024) knots 0 0 0 1 2 2 2
  spline S426 degree 2 poles (10.4039, 63.7024) (10.4039, 63.9444) (10.2071, 64.1173) (10.0688, 64.1173) knots 0 0 0 1 2 2 2
  spline S427 degree 2 poles (10.0688, 64.1173) (10.013, 64.1173) (9.9571, 64.1013) knots 0 0 0 1 1 1
  spline S428 degree 2 poles (9.9571, 64.1013) (9.9013, 64.0854) (9.8481, 64.0535) knots 0 0 0 1 1 1
  spline S429 degree 2 poles (9.8481, 64.0535) (9.8055, 64.0269) (9.7683, 63.9843) knots 0 0 0 1 1 1
  spline S430 degree 2 poles (9.7683, 63.9843) (9.7284, 63.9418) (9.6965, 63.878) knots 0 0 0 1 1 1
  spline S431 degree 2 poles (9.6965, 63.878) (9.6593, 63.8008) (9.6406, 63.7131) knots 0 0 0 1 1 1
  spline S432 degree 2 poles (9.6406, 63.7131) (9.6167, 63.5907) (9.6007, 63.4019) knots 0 0 0 1 1 1
  spline S433 degree 2 poles (9.6007, 63.4019) (9.5928, 63.2663) (9.5768, 62.9286) knots 0 0 0 1 1 1
  line L111 (9.5768, 62.9286) -> (9.5609, 62.4445)
  spline S434 degree 2 poles (9.5609, 62.4445) (9.2603, 62.4499) (9.0662, 62.4499) knots 0 0 0 1 1 1
  spline S435 degree 2 poles (9.0662, 62.4499) (8.8508, 62.4499) (8.6327, 62.4445) knots 0 0 0 1 1 1
  spline S436 degree 2 poles (8.6327, 62.4445) (8.6859, 63.0349) (8.7471, 64.096) (8.763, 64.8141) knots 0 0 0 1 2 2 2
  spline S437 degree 2 poles (5.9414, 64.1146) (5.9707, 64.2529) (6.0584, 64.7875) knots 0 0 0 1 1 1
  spline S438 degree 2 poles (6.0584, 64.7875) (6.327, 64.8407) (6.694, 64.8752) (6.8828, 64.8752) knots 0 0 0 1 2 2 2
  spline S439 degree 2 poles (6.8828, 64.8752) (7.1594, 64.8752) (7.6222, 64.7981) (7.9599, 64.604) (8.1859, 64.3141) (8.3056, 63.9152) (8.3056, 63.7024) knots 0 0 0 1 2 3 4 5 5 5
  spline S440 degree 2 poles (8.3056, 63.7024) (8.3056, 63.4072) (8.0689, 62.8381) (7.694, 62.519) (7.2073, 62.3834) (6.952, 62.3834) knots 0 0 0 1 2 3 4 4 4
  spline S441 degree 2 poles (6.952, 62.3834) (6.6887, 62.3834) (6.2074, 62.5057) (5.8723, 62.8115) (5.7313, 63.1972) (5.7313, 63.4205) knots 0 0 0 1 2 3 4 4 4
  spline S442 degree 2 poles (5.7313, 63.4205) (5.7313, 63.5535) (5.7606, 63.7157) knots 0 0 0 1 1 1
  line L112 (5.7606, 63.7157) -> (7.3881, 63.7184)
  spline S443 degree 2 poles (7.3881, 63.7184) (7.3908, 63.7556) (7.3908, 63.7849) knots 0 0 0 1 1 1
  spline S444 degree 2 poles (7.3908, 63.7849) (7.3908, 64.0349) (7.0318, 64.2715) (6.7765, 64.2715) knots 0 0 0 1 2 2 2
  spline S445 degree 2 poles (6.7765, 64.2715) (6.6222, 64.2715) (6.2286, 64.1997) (5.9414, 64.1146) knots 0 0 0 1 2 2 2
  line L113 (7.3695, 63.362) -> (6.6036, 63.362)
  spline S446 degree 2 poles (6.6036, 63.362) (6.6009, 63.3221) (6.6009, 63.2956) knots 0 0 0 1 1 1
  spline S447 degree 2 poles (6.6009, 63.2956) (6.6009, 63.1732) (6.686, 63.003) (6.8483, 62.9232) (6.9467, 62.9232) knots 0 0 0 1 2 3 3 3
  spline S448 degree 2 poles (6.9467, 62.9232) (7.0158, 62.9232) (7.1461, 62.9684) (7.2525, 63.0535) (7.3216, 63.1652) (7.3536, 63.269) (7.3695, 63.362) knots 0 0 0 1 2 3 4 5 5 5
  line L114 (5.4308, 64.8141) -> (5.3883, 64.3141)
  line L115 (5.3883, 64.3141) -> (5.3005, 62.5775)
  line L116 (5.3005, 62.5775) -> (5.2739, 61.6441)
  spline S449 degree 2 poles (5.2739, 61.6441) (4.9521, 61.6494) (4.7899, 61.6494) knots 0 0 0 1 1 1
  spline S450 degree 2 poles (4.7899, 61.6494) (4.5771, 61.6494) (4.3218, 61.6441) knots 0 0 0 1 1 1
  line L117 (4.3218, 61.6441) -> (4.375, 62.3568)
  line L118 (4.375, 62.3568) -> (4.4601, 64.112)
  line L119 (4.4601, 64.112) -> (4.4788, 64.8141)
  spline S451 degree 2 poles (4.4788, 64.8141) (4.7261, 64.8114) (4.9255, 64.8114) knots 0 0 0 1 1 1
  line L120 (4.9255, 64.8114) -> (5.4308, 64.8141)
  spline S452 degree 2 poles (1.6545, 64.1146) (1.6837, 64.2529) (1.7715, 64.7875) knots 0 0 0 1 1 1
  spline S453 degree 2 poles (1.7715, 64.7875) (2.0401, 64.8407) (2.4071, 64.8752) (2.5959, 64.8752) knots 0 0 0 1 2 2 2
  spline S454 degree 2 poles (2.5959, 64.8752) (2.8725, 64.8752) (3.3352, 64.7981) (3.673, 64.604) (3.899, 64.3141) (4.0187, 63.9152) (4.0187, 63.7024) knots 0 0 0 1 2 3 4 5 5 5
  spline S455 degree 2 poles (4.0187, 63.7024) (4.0187, 63.4072) (3.782, 62.8381) (3.407, 62.519) (2.9203, 62.3834) (2.665, 62.3834) knots 0 0 0 1 2 3 4 4 4
  spline S456 degree 2 poles (2.665, 62.3834) (2.4018, 62.3834) (1.9204, 62.5057) (1.5853, 62.8115) (1.4444, 63.1972) (1.4444, 63.4205) knots 0 0 0 1 2 3 4 4 4
  spline S457 degree 2 poles (1.4444, 63.4205) (1.4444, 63.5535) (1.4736, 63.7157) knots 0 0 0 1 1 1
  line L121 (1.4736, 63.7157) -> (3.1012, 63.7184)
  spline S458 degree 2 poles (3.1012, 63.7184) (3.1038, 63.7556) (3.1038, 63.7849) knots 0 0 0 1 1 1
  spline S459 degree 2 poles (3.1038, 63.7849) (3.1038, 64.0349) (2.7448, 64.2715) (2.4895, 64.2715) knots 0 0 0 1 2 2 2
  spline S460 degree 2 poles (2.4895, 64.2715) (2.3353, 64.2715) (1.9417, 64.1997) (1.6545, 64.1146) knots 0 0 0 1 2 2 2
  line L122 (3.0826, 63.362) -> (2.3167, 63.362)
  spline S461 degree 2 poles (2.3167, 63.362) (2.314, 63.3221) (2.314, 63.2956) knots 0 0 0 1 1 1
  spline S462 degree 2 poles (2.314, 63.2956) (2.314, 63.1732) (2.3991, 63.003) (2.5613, 62.9232) (2.6597, 62.9232) knots 0 0 0 1 2 3 3 3
  spline S463 degree 2 poles (2.6597, 62.9232) (2.7289, 62.9232) (2.8592, 62.9684) (2.9656, 63.0535) (3.0347, 63.1652) (3.0666, 63.269) (3.0826, 63.362) knots 0 0 0 1 2 3 4 5 5 5
  point P0 (0, 0)
  constraints: 3 other
extrude "Estrusione5" cut sketch "Schizzo6" against normal blind 1
